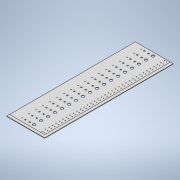
# Autodesk Inventor part: linerFlat
Saved by Autodesk Inventor 2021.2 (Build 252289000, 289)
## iProperties
Created: 2021-06-06
Part Number: linerFlat
Material: Generic
Document SubType Name: Modeling
Designer: Ryan
Density: 1 g/cm^3
Appearance: Default
Author: Ryan
Autodesk Inventor part; units mm, degrees
ref_plane "YZ Plane" through (0, 0, 0) normal (1, 0, 0) x (0, 1, 0)
ref_plane "XZ Plane" through (0, 0, 0) normal (0, 1, 0) x (-1, 0, 0)
ref_plane "XY Plane" through (0, 0, 0) normal (0, 0, 1) x (1, 0, 0)
sketch "Sketch1" plane through (0, 0, 0) normal (0, 0, 1) x (1, 0, 0)
  line L0 (0, 0) -> (82.55, 0)
  line L1 (82.55, 0) -> (82.55, 0.7937)
  line L2 (82.55, 0.7937) -> (0, 0.7937)
  line L3 (0, 0.7937) -> (0, 0)
  dimension "d0" = 82.55
  dimension "d1" = 0.7937
  constraints: 8 end point, 2 parallel, 1 horizontal, 1 perpendicular
  measures "d0" distance of L2.end L1.end
  measures "d1" distance of L0.end L1.end
extrude "Extrusion1" add sketch "Sketch1" along normal blind 295.275
sketch "Sketch2" plane through (0, 0.7937, 0) normal (0, 1, 0) x (1, 0, 0)
  line L0 (82.55, 0) -> (82.55, -295.275) projected
  circle A0 centre (49.53, -8.2021) radius 3.175
  circle A1 centre (39.37, -8.2021) radius 1.5875
  circle A2 centre (29.21, -8.2021) radius 1.5875
  circle A3 centre (21.59, -8.2021) radius 0.7937
  line L1 (82.55, 0) -> (0, 0) projected
  dimension "d8" = 6.35
  dimension "d9" = 3.175
  dimension "d10" = 3.175
  dimension "d11" = 1.5875
  dimension "d12" = 33.02
  dimension "d13" = 43.18
  dimension "d14" = 53.34
  dimension "d16" = 7.62
  dimension "d19" = 8.2021
  dimension "d20" = 8.2021
  dimension "d21" = 8.2021
  dimension "d22" = 8.2021
  constraints: 4 centre point
  measures "d8" diameter of A0
  measures "d9" diameter of A1
  measures "d10" diameter of A2
  measures "d11" diameter of A3
  measures "d12" distance from line of A0.centre L0
  measures "d13" distance from line of L0 A1.centre
  measures "d14" distance from line of A2.centre L0
  measures "d16" distance of A3.centre A2.centre
  measures "d19" distance from line of A0.centre L1
  measures "d20" distance from line of L1 A1.centre
  measures "d21" distance from line of L1 A2.centre
  measures "d22" distance from line of L1 A3.centre
extrude "Extrusion2" cut sketch "Sketch2" against normal through all
pattern_linear "Rectangular Pattern1" count 18 spacing 16.4042 along (0, 0, 1) of "Extrusion2"
sketch "Sketch3" plane through (0, 0.7937, 0) normal (0, 1, 0) x (1, 0, 0)
  circle A0 centre (77.47, -4.101) radius 0.7938
  circle A1 centre (72.39, -4.101) radius 0.7937
  line L0 (82.55, 0) -> (82.55, -295.275) projected
  line L1 (82.55, 0) -> (0, 0) projected
  dimension "d28" = 1.5875
  dimension "d29" = 1.5875
  dimension "d30" = 5.08
  dimension "d31" = 10.16
  dimension "d32" = 4.101
  dimension "d33" = 4.101
  constraints: 2 centre point
  measures "d28" diameter of A0
  measures "d29" diameter of A1
  measures "d30" distance from line of L0 A0.centre
  measures "d31" distance from line of L0 A1.centre
  measures "d32" distance from line of L1 A0.centre
  measures "d33" distance from line of L1 A1.centre
extrude "Extrusion3" cut sketch "Sketch3" against normal through all
pattern_linear "Rectangular Pattern2" count 36 spacing 8.2021 along (0, 0, 1) of "Extrusion3"
sketch "Sketch4" plane through (0, 0, 295.275) normal (0, 0, 1) x (1, 0, 0)
  line L0 (0, 0) -> (82.55, 0) projected
  line L1 (82.55, 0.7937) -> (0, 0.7937) projected
  line L2 (0, 0) -> (82.55, 0)
  line L3 (82.55, 0) -> (82.55, 0.7937)
  line L4 (82.55, 0.7937) -> (0, 0.7937)
  line L5 (0, 0.7937) -> (0, 0)
  constraints: 8 end point, 2 parallel, 1 horizontal, 1 perpendicular
extrude "Extrusion4" add sketch "Sketch4" along normal blind 6.35
sketch "Sketch5" plane through (82.55, 0.7937, 301.625) normal (1, 0, 0) x (0, 0, -1)
  line L0 (301.625, -0.7937) -> (0, -0.7937) projected
  line L1 (301.625, -0.7937) -> (301.625, 0) projected
  line L2 (0, -0.7937) -> (301.625, -0.7937)
  line L3 (301.625, -0.7937) -> (301.625, 0)
  line L4 (301.625, 0) -> (0, 0)
  line L5 (0, 0) -> (0, -0.7937)
  constraints: 8 end point, 2 parallel, 1 horizontal, 1 perpendicular
extrude "Extrusion5" add sketch "Sketch5" along normal blind 6.35
sketch "Sketch6" plane through (0, 0.7937, 301.625) normal (0, 1, 0) x (1, 0, 0)
  line L0 (88.9, 301.625) -> (88.9, 0) projected
  line L1 (0, 0) -> (88.9, 0) projected
  line L2 (88.9, 301.625) -> (82.55, 301.625)
  line L3 (82.55, 0) -> (88.9, 0)
  line L4 (88.9, 0) -> (88.9, 301.625)
  line L5 (0, 301.625) -> (0, 0) projected
  line L6 (88.9, 0) -> (0, 0)
  line L7 (0, 0) -> (0, 6.35)
  line L8 (88.9, 6.35) -> (88.9, 0)
  line L9 (82.55, 301.625) -> (82.55, 6.35)
  line L10 (82.55, 6.35) -> (0, 6.35)
  dimension "d43" = 6.35
  dimension "d44" = 6.35
  constraints: 16 end point, 2 horizontal, 2 parallel, 2 perpendicular, 2 point on line
  measures "d43" distance of L3.end L3.start
  measures "d44" distance of L6.end L7.end
extrude "Extrusion6" add sketch "Sketch6" along normal blind 0.3969
body "Solid1"
